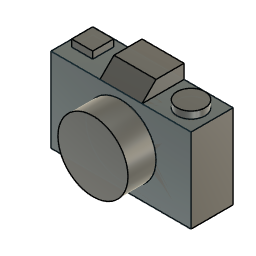
EDM EXP 2.1 v1 (Autodesk Fusion 360 design; units mm, degrees)
Autodesk Fusion 360 part; units mm, degrees
sketch "Sketch1" plane through (0, 0, 0) normal (0, 1, 0) x (1, 0, 0)
  line L0 (50, 30) -> (-50, 30)
  line L1 (-50, 30) -> (-50, -30)
  line L2 (-50, -30) -> (50, -30)
  line L3 (50, -30) -> (50, 30)
  line L4 (50, 30) -> (-50, -30) construction
  line L5 (-50, 30) -> (50, -30) construction
  dimension "d1" = 100
  dimension "d2" = 60
  constraint horizontal L0
  constraint perpendicular L0 L1
  constraint parallel L0 L2
  constraint parallel L1 L3
  constraint coincident L4 origin
  constraint coincident L5 origin
  measures "d1" distance of L1.end L2.end
  measures "d2" distance of L0.end L1.end
extrude "Extrude1" add sketch "Sketch1" along normal blind 30
sketch "Sketch2" plane through (0, 0, 0) normal (0, 1, 0) x (1, 0, 0)
  circle A0 centre (0, 0) radius 25
  dimension "d5" = 50
  constraint coincident A0.centre origin
  measures "d5" diameter of A0
extrude "Extrude2" add sketch "Sketch2" against normal blind 20
sketch "Sketch3" plane through (0, 0, 0) normal (0, -1, 0) x (1, 0, 0)
  circle A0 centre (0, 0) radius 25
  line L0 (50, -30) -> (50, 30)
  line L1 (50, 30) -> (-50, 30)
  line L2 (-50, 30) -> (-50, -30)
  line L3 (-50, -30) -> (50, -30)
sketch "Sketch4" plane through (0, 0, 30) normal (0, 0, 1) x (-1, 0, 0)
  line L0 (50, 0) -> (-50, 0)
  line L1 (-50, 0) -> (-50, -30)
  line L2 (-50, -30) -> (50, -30)
  line L3 (50, -30) -> (50, 0)
  circle A0 centre (-35, -15) radius 10
  line L4 (42.5777, -25.1555) -> (27.5777, -25.1555)
  line L5 (27.5777, -25.1555) -> (27.5777, -10.1555)
  line L6 (27.5777, -10.1555) -> (42.5777, -10.1555)
  line L7 (42.5777, -10.1555) -> (42.5777, -25.1555)
  dimension "d8" = 20
  dimension "d9" = 15
  dimension "d10" = 15
  constraint horizontal L4
  constraint vertical L5
  constraint horizontal L6
  constraint vertical L7
  measures "d8" diameter of A0
  measures "d9" distance of L4.start L4.end
  measures "d10" distance of L4.start L6.end
extrude "Extrude3" add sketch "Sketch4" along normal blind 5 contours A0
sketch "Sketch5" plane through (0, 0, 30) normal (0, 0, 1) x (-1, 0, 0)
  circle A0 centre (-35, -15) radius 10
  line L0 (50, 0) -> (-50, 0)
  line L1 (-50, 0) -> (-50, -30)
  line L2 (-50, -30) -> (50, -30)
  line L3 (50, -30) -> (50, 0)
  line L4 (45.1493, -24.9291) -> (30.1493, -24.9291)
  line L5 (30.1493, -24.9291) -> (30.1493, -9.9291)
  line L6 (30.1493, -9.9291) -> (45.1493, -9.9291)
  line L7 (45.1493, -9.9291) -> (45.1493, -24.9291)
  dimension "d13" = 15
  dimension "d14" = 15
  constraint horizontal L4
  constraint vertical L5
  constraint horizontal L6
  constraint vertical L7
  measures "d13" distance of L4.start L4.end
  measures "d14" distance of L4.start L6.end
extrude "Extrude4" add sketch "Sketch5" along normal blind 5 contours L4 L5 L6 L7
sketch "Sketch6" plane through (0, 0, 30) normal (0, 0, 1) x (-1, 0, 0)
  line L0 (45.1493, -9.9291) -> (45.1493, -24.9291)
  line L1 (45.1493, -24.9291) -> (30.1493, -24.9291)
  line L2 (30.1493, -24.9291) -> (30.1493, -9.9291)
  line L3 (30.1493, -9.9291) -> (45.1493, -9.9291)
  circle A0 centre (-35, -15) radius 10
  line L4 (50, 0) -> (-50, 0)
  line L5 (-50, 0) -> (-50, -30)
  line L6 (-50, -30) -> (50, -30)
  line L7 (50, -30) -> (50, 0)
box "BoxPrimitive1" add length 30 width 30 height 10 placed x (0, -1, 0) y (1, 0, 0) z (0, 0, 1) at (-15, 30, 30)
chamfer "Chamfer1" distance 10 angle 45 1 edges at (0, 0, 40)
